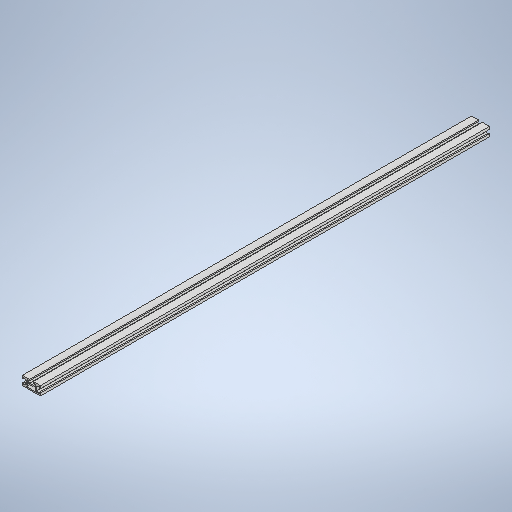
# Autodesk Inventor part: Part1
Saved by Autodesk Inventor 2025.2 (Build 292293000, 293)
## iProperties
Created: 2025-04-03
Part Number: Part1
Material: Generic
Document SubType Name: Modeling
Designer: kenne
Density: 1 g/cm^3
Appearance: Default
Author: kenne
Autodesk Inventor part; units mm, degrees
ref_plane "YZ Plane" through (0, 0, 0) normal (1, 0, 0) x (0, 1, 0)
ref_plane "XZ Plane" through (0, 0, 0) normal (0, 1, 0) x (-1, 0, 0)
ref_plane "XY Plane" through (0, 0, 0) normal (0, 0, 1) x (1, 0, 0)
sketch "Sketch1" plane through (0, 0, 0) normal (0, 0, 1) x (1, 0, 0)
  line L0 (-15, 7.5) -> (15, 7.5) construction
  line L1 (0, 10.5) -> (0, -10.5) projected
  line L2 (-15, 7.5) -> (-15, -7.5) construction
  line L3 (-15, 3.1) -> (-15, -3.1) construction
  line L4 (-15, 7.5) -> (-15, 3.1)
  line L5 (-15, 7.5) -> (-3.1, 7.5)
  line L6 (-15, 3.1) -> (-13, 3.1)
  line L7 (-3.1, 5.5) -> (-3.1, 7.5)
  line L8 (-13, 3.1) -> (-13, 5.5)
  line L9 (-15, 3.1) -> (-9, 3.1) construction
  line L10 (-13, 5.5) -> (-9, 3.1)
  line L11 (-9, 0) -> (-9, 3.1)
  line L12 (-21, 0) -> (21, 0) projected
  line L13 (-9, 0) -> (-9, -3.1)
  line L14 (-9, -3.1) -> (-13, -5.5)
  line L15 (-13, -5.5) -> (-13, -3.1)
  line L16 (-13, -3.1) -> (-15, -3.1)
  line L17 (-15, -3.1) -> (-15, -7.5)
  line L18 (-15, -7.5) -> (0, -7.5)
  line L19 (0, -7.5) -> (0, -5.5)
  line L20 (0, -5.5) -> (-9.1127, -5.5)
  line L21 (-9.1127, -5.5) -> (-7, -4.2324)
  line L22 (-7, -4.2324) -> (-7, 3.2725)
  line L23 (0, 0) -> (-3.1, 0)
  line L24 (-7, 3.2725) -> (-3.1, 0)
  line L25 (-3.1, 5.5) -> (-7, 5.5)
  line L26 (-7, 5.5) -> (-3.1, 1.9884)
  line L27 (-3.1, 1.9884) -> (0, 1.9884)
  line L28 (0, 1.9884) -> (0, 0)
  point P0 (0, 7.5)
  point P1 (-15, 0)
  dimension "d0" = 7.5
  dimension "d1" = 30
  dimension "d2" = 15
  dimension "d3" = 6.2
  dimension "d4" = 3.1
  dimension "d5" = 2
  dimension "d6" = 2.4
  dimension "d7" = 6
  dimension "d8" = 3.1
  dimension "d9" = 2
  dimension "d10" = 2
  dimension "d11" = 2
  dimension "d12" = 50
  dimension "d13" = 2
  constraints: 54 end point, 8 point on line, 7 horizontal, 7 vertical, 4 vertical alignment, 3 collinear, 3 equal length, 3 midpoint, 1 parallel
  measures "d0" distance from line of L0 L23.start
  measures "d1" distance of L0.start L0.end
  measures "d2" distance of L0.start L2.end
  measures "d3" distance of L3.start L3.end
  measures "d4" distance from line of L1 L5.end
  measures "d5" distance of L3.start L6.end
  measures "d6" distance of L6.end L8.end
  measures "d7" distance of L3.start L9.end
  measures "d8" distance of L11.start L13.end
  measures "d9" distance of L18.end L19.end
  measures "d10" distance between parallel lines of L21 L14
  measures "d11" distance between parallel lines of L22 L11
  measures "d12" angle of L22 L24
  measures "d13" angle of L24 L26
extrude "Extrusion1" add sketch "Sketch1" along normal mid plane 750 contours L1 L12 L24 L22 L11 L10 L8 L6 L4 L5 L7 L25 L26 L27 | L1 L18 L17 L16 L15 L14 L13 L12 L22 L21 L20
mirror "Mirror1" about plane through (0, 0, 0) normal (1, 0, 0) of "Extrusion1"
body "Solid1"
